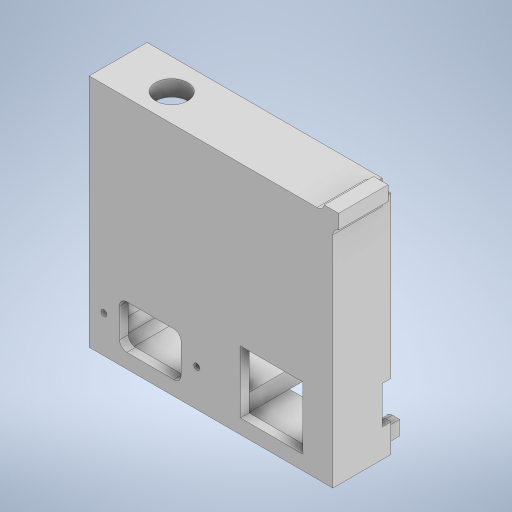
# Autodesk Inventor part: bottom
Saved by Autodesk Inventor 2023 (Build 270158000, 158)
## iProperties
Created: 2022-04-19
Part Number: bottom
Material: Generic
Document SubType Name: Modeling
Designer: cooki
Density: 1 g/cm^3
Appearance: Default
Author: cooki
## iProperties of the stored document bottom_3DPrint.ipt
Created: 2022-04-21
Part Number: bottom_3DPrint
Material: Generic
Document SubType Name: Modeling
Designer: cooki
Density: 1 g/cm^3
Appearance: Default
Author: cooki
Autodesk Inventor part; units mm, degrees
(part 1 of 2)
ref_plane "YZ Plane" through (0, 0, 0) normal (1, 0, 0) x (0, 1, 0)
ref_plane "XZ Plane" through (0, 0, 0) normal (0, 1, 0) x (-1, 0, 0)
ref_plane "XY Plane" through (0, 0, 0) normal (0, 0, 1) x (1, 0, 0)
sketch "Sketch1" plane through (0, 0, 0) normal (0, 0, 1) x (1, 0, 0)
  line L0 (53.34, -10.795) -> (50.8, -10.795) projected
  line L1 (50.8, -48.895) -> (50.8, -10.795) projected
  line L2 (-50.8, -48.895) -> (50.8, -48.895) projected
  line L3 (-50.8, 48.895) -> (-50.8, -48.895) projected
  line L4 (-49.3242, 48.895) -> (-50.8, 48.895) projected
  line L5 (-49.3242, 48.895) -> (-49.3242, 51.435) projected
  line L6 (-53.34, 51.435) -> (-49.3242, 51.435) projected
  line L7 (-53.34, -51.435) -> (-53.34, 51.435) projected
  line L8 (53.34, -51.435) -> (-53.34, -51.435) projected
  line L9 (53.34, -10.795) -> (53.34, -51.435) projected
  line L10 (-49.3242, 48.895) -> (50.8, 48.895)
  line L11 (-49.3242, 51.435) -> (53.34, 51.435)
  line L12 (50.8, -10.795) -> (50.8, 48.895)
  line L13 (53.34, -10.795) -> (53.34, 51.435)
  point P0 (0, 0)
  constraints: 8 end point, 2 horizontal, 2 vertical
extrude "Extrusion1" add sketch "Sketch1" along normal blind 19.05 contours L9 L8 L7 L6 L5 L4 L3 L2 L1 L0 | L0 L12 L10 L5 L11 L13
sketch "Sketch2" plane through (0, 0, 19.05) normal (0, 0, 1) x (1, 0, 0)
  line L0 (-53.34, 51.435) -> (-53.34, -51.435) projected
  line L1 (-53.34, -51.435) -> (53.34, -51.435) projected
  line L2 (-53.34, 51.435) -> (53.34, 51.435)
  line L3 (53.34, 51.435) -> (53.34, -51.435)
  line L4 (53.34, -51.435) -> (-53.34, -51.435)
  line L5 (-53.34, -51.435) -> (-53.34, 51.435)
  point P0 (0, 0)
  constraints: 8 end point, 2 parallel, 1 horizontal, 1 perpendicular
extrude "Extrusion2" add sketch "Sketch2" along normal blind 3.81
sketch "Sketch3" plane through (0, 0, 22.86) normal (0, 0, 1) x (1, 0, 0)
  line L0 (49.53, -22.225) -> (-49.53, -22.225) projected
  line L1 (0, -22.225) -> (0, -48.895)
  line L2 (50.8, -48.895) -> (-50.8, -48.895) projected
  line L3 (0, -35.56) -> (53.34, -35.56)
  line L4 (53.34, -51.435) -> (53.34, 51.435) projected
  line L5 (26.67, -35.56) -> (26.67, -45.085)
  line L6 (26.67, -45.085) -> (36.83, -45.085)
  line L7 (40.005, -45.085) -> (16.256, -45.085)
  line L8 (13.081, -41.91) -> (13.081, -29.083)
  line L9 (16.256, -25.908) -> (36.83, -25.908)
  line L10 (40.005, -29.083) -> (40.005, -41.91)
  arc A0 (36.83, -45.085) -> (40.005, -41.91) centre (36.83, -41.91) ccw
  arc A1 (13.081, -41.91) -> (16.256, -45.085) centre (16.256, -41.91) ccw
  arc A2 (40.005, -29.083) -> (36.83, -25.908) centre (36.83, -29.083) ccw
  arc A3 (16.256, -25.908) -> (13.081, -29.083) centre (16.256, -29.083) ccw
  line L11 (-26.67, -45.085) -> (-36.83, -45.085)
  line L12 (-40.005, -45.085) -> (-16.256, -45.085)
  line L13 (-13.081, -41.91) -> (-13.081, -29.083)
  line L14 (-16.256, -25.908) -> (-36.83, -25.908)
  line L15 (-40.005, -29.083) -> (-40.005, -41.91)
  arc A4 (-40.005, -41.91) -> (-36.83, -45.085) centre (-36.83, -41.91) ccw
  arc A5 (-16.256, -45.085) -> (-13.081, -41.91) centre (-16.256, -41.91) ccw
  arc A6 (-36.83, -25.908) -> (-40.005, -29.083) centre (-36.83, -29.083) ccw
  arc A7 (-13.081, -29.083) -> (-16.256, -25.908) centre (-16.256, -29.083) ccw
  point P0 (0, 0)
  point P1 (13.081, -25.908)
  point P2 (13.081, -45.085)
  point P3 (40.005, -25.908)
  dimension "d4" = 9.525
  dimension "d5" = 13.335
  dimension "d6" = 26.924
  dimension "d7" = 19.177
  dimension "d8" = 3.175
  constraints: 26 end point, 16 point on circle, 14 symmetric about line, 11 point on line, 8 centre point, 8 tangent, 4 midpoint, 3 equal radius, 2 horizontal, 2 parallel, 2 perpendicular, 1 vertical, 4 other
  measures "d4" distance of L5.start L5.end
  measures "d5" distance of L5.end L7.start
  measures "d6" distance of point (13.081, -25.908) point (40.005, -25.908)
  measures "d7" distance of point (13.081, -45.085) point (13.081, -25.908)
  measures "d8" radius of A0
extrude "Extrusion3" cut sketch "Sketch3" against normal blind 3.81
sketch "Sketch4" plane through (0, 0, 22.86) normal (0, 0, 1) x (1, 0, 0)
  line L0 (50.8, -48.895) -> (50.8, 48.895)
  line L1 (50.8, 48.895) -> (-50.8, 48.895)
  line L2 (-50.8, 48.895) -> (-50.8, -48.895)
  line L3 (-50.8, -48.895) -> (50.8, -48.895)
  line L4 (-16.256, -45.085) -> (-36.83, -45.085)
  arc A0 (-40.005, -41.91) -> (-36.83, -45.085) centre (-36.83, -41.91) ccw
  line L5 (-40.005, -41.91) -> (-40.005, -29.083)
  arc A1 (-36.83, -25.908) -> (-40.005, -29.083) centre (-36.83, -29.083) ccw
  line L6 (-36.83, -25.908) -> (-16.256, -25.908)
  arc A2 (-13.081, -29.083) -> (-16.256, -25.908) centre (-16.256, -29.083) ccw
  line L7 (-13.081, -29.083) -> (-13.081, -41.91)
  arc A3 (-16.256, -45.085) -> (-13.081, -41.91) centre (-16.256, -41.91) ccw
  arc A4 (13.081, -41.91) -> (16.256, -45.085) centre (16.256, -41.91) ccw
  line L8 (13.081, -41.91) -> (13.081, -29.083)
  arc A5 (16.256, -25.908) -> (13.081, -29.083) centre (16.256, -29.083) ccw
  line L9 (16.256, -25.908) -> (36.83, -25.908)
  arc A6 (40.005, -29.083) -> (36.83, -25.908) centre (36.83, -29.083) ccw
  line L10 (40.005, -29.083) -> (40.005, -41.91)
  arc A7 (36.83, -45.085) -> (40.005, -41.91) centre (36.83, -41.91) ccw
  line L11 (36.83, -45.085) -> (16.256, -45.085)
  line L12 (53.34, 51.435) -> (-53.34, 51.435)
  line L13 (-53.34, 51.435) -> (-53.34, -51.435)
  line L14 (-53.34, -51.435) -> (53.34, -51.435)
  line L15 (53.34, -51.435) -> (53.34, 51.435)
  line L16 (26.543, -35.179) -> (6.223, -35.179)
  line L17 (6.223, -35.179) -> (46.863, -35.179)
  line L18 (50.8, -48.895) -> (-50.8, -48.895)
  line L19 (0, -48.895) -> (0, -20.9574)
  circle A8 centre (6.223, -35.179) radius 1.27
  circle A9 centre (46.863, -35.179) radius 1.27
  circle A10 centre (-6.223, -35.179) radius 1.27
  circle A11 centre (-46.863, -35.179) radius 1.27
  spline S0 degree 3 poles (5.1978, -26.6049) (5.0531, -26.6049) (4.9129, -26.5796) (4.651, -26.4704) (4.5374, -26.3925) (4.3198, -26.1853) (4.2361, -26.0666) (4.1512, -25.8725) (4.1298, -25.8046) (4.101, -25.6619) (4.0942, -25.5884) (4.0942, -25.5145) knots 0 0 0 0 0.236242 0.236242 0.463278 0.463278 0.726641 0.726641 0.861093 0.861093 1 1 1 1
  spline S1 degree 3 poles (4.0942, -25.5145) (4.0942, -25.3737) (4.1187, -25.2372) (4.2245, -24.9834) (4.2996, -24.8739) (4.4749, -24.6902) (4.597, -24.585) (4.8289, -24.4831) (4.899, -24.4609) (5.046, -24.4311) (5.1217, -24.424) (5.1978, -24.424) knots 0 0 0 0 0.28445 0.28445 0.555633 0.555633 0.797647 0.797647 0.897296 0.897296 1 1 1 1
  spline S2 degree 3 poles (5.1978, -24.424) (5.3475, -24.424) (5.4929, -24.4496) (5.7606, -24.561) (5.875, -24.6392) (6.0718, -24.8281) (6.1657, -24.9455) (6.2583, -25.1585) (6.2794, -25.226) (6.3079, -25.3679) (6.3146, -25.441) (6.3146, -25.5145) knots 0 0 0 0 0.276403 0.276403 0.535347 0.535347 0.780114 0.780114 0.888262 0.888262 1 1 1 1
  spline S3 degree 3 poles (6.3146, -25.5145) (6.3146, -25.6552) (6.2901, -25.7917) (6.1843, -26.0455) (6.1092, -26.1551) (5.9462, -26.326) (5.8257, -26.4366) (5.5805, -26.5444) (5.5081, -26.567) (5.3558, -26.5978) (5.277, -26.6049) (5.1978, -26.6049) knots 0 0 0 0 0.306185 0.306185 0.598089 0.598089 0.819962 0.819962 0.908282 0.908282 1 1 1 1
  spline S4 degree 3 poles (9.8618, -39.2173) (9.7254, -39.2173) (9.5913, -39.1958) (9.33, -39.0883) (9.2363, -39.0116) (9.0945, -38.8721) (9.0324, -38.7816) (8.9368, -38.5537) (8.9159, -38.4198) (8.9159, -38.2846) knots 0 0 0 0 0.195595 0.195595 0.405153 0.405153 0.67435 0.67435 1 1 1 1
  spline S5 degree 3 poles (8.9159, -38.2846) (8.9159, -37.4855) (9.0782, -36.5199) (9.2325, -35.5792) (9.3231, -34.8494) (9.3231, -34.2512) knots 0 0 0 0 0.239723 0.239723 0.894859 0.894859 0.894859 0.894859
  line L20 (9.3231, -34.2512) -> (9.31, -33.371)
  line L21 (9.31, -33.371) -> (9.31, -32.425)
  spline S6 degree 3 poles (9.31, -32.425) (9.3214, -31.9255) (9.3575, -31.3944) (9.5041, -30.5323) (9.6012, -30.1386) (9.7567, -29.7974) knots 0 0 0 0 0.572323 0.572323 1 1 1 1
  spline S7 degree 3 poles (9.7567, -29.7974) (9.8824, -29.5153) (10.0496, -29.255) (10.4599, -28.8616) (10.6752, -28.7258) (11.2164, -28.5155) (11.5377, -28.4705) (11.8588, -28.4705) knots 0 0 0 0 0.34729 0.34729 0.638954 0.638954 1 1 1 1
  spline S8 degree 3 poles (11.8588, -28.4705) (12.2099, -28.4705) (12.5487, -28.5408) (13.2841, -28.8321) (13.657, -29.0802) (14.4056, -29.7206) (14.7781, -30.1487) (15.1038, -30.5857) knots 0 0 0 0 0.262666 0.262666 0.591662 0.591662 1 1 1 1
  line L22 (15.1038, -30.5857) -> (15.1301, -29.4821)
  spline S9 degree 3 poles (15.1301, -29.4821) (15.1473, -29.2515) (15.1886, -29.0015) (15.3312, -28.672) (15.3984, -28.5628) (15.5607, -28.4025) (15.6433, -28.3479) (15.8489, -28.2651) (15.9686, -28.2472) (16.0892, -28.2472) knots 0 0 0 0 0.399692 0.399692 0.618402 0.618402 0.792341 0.792341 1 1 1 1
  spline S10 degree 3 poles (16.0892, -28.2472) (16.221, -28.2472) (16.3498, -28.2687) (16.6015, -28.3727) (16.6969, -28.4489) (16.8417, -28.5901) (16.9052, -28.6808) (16.9741, -28.8429) (16.992, -28.9033) (17.0164, -29.0319) (17.022, -29.0993) (17.022, -29.1668) knots 0 0 0 0 0.201212 0.201212 0.415858 0.415858 0.686307 0.686307 0.838093 0.838093 1 1 1 1
  spline S11 degree 3 poles (17.022, -29.1668) (17.022, -29.4784) (16.9959, -29.9443) (16.9753, -30.3191) (16.9563, -30.7049) (16.9563, -30.9667) knots 0 0 0 0 0.326745 0.326745 1 1 1 1
  spline S12 degree 3 poles (16.9563, -30.9667) (16.9563, -31.9695) (17.0606, -33.3007) (17.1487, -34.4506) (17.219, -35.5256) (17.219, -36.3401) knots 0 0 0 0 0.30083 0.30083 0.980723 0.980723 0.980723 0.980723
  spline S13 degree 3 poles (17.219, -36.3401) (17.219, -36.6382) (17.172, -37.0783) (17.1299, -37.4813) (17.1008, -37.8136) (17.1008, -38.0481) knots 0 0 0 0 0.287253 0.287253 1 1 1 1
  spline S14 degree 3 poles (17.1008, -38.0481) (17.1008, -38.1867) (17.0799, -38.3241) (16.9761, -38.579) (16.9052, -38.6703) (16.7594, -38.8172) (16.6678, -38.8798) (16.442, -38.9735) (16.3125, -38.994) (16.1811, -38.994) knots 0 0 0 0 0.220047 0.220047 0.436643 0.436643 0.697196 0.697196 1 1 1 1
  spline S15 degree 3 poles (16.1811, -38.994) (16.0491, -38.994) (15.9191, -38.9733) (15.6914, -38.8797) (15.5984, -38.8171) (15.452, -38.6732) (15.3779, -38.5821) (15.2701, -38.3255) (15.2484, -38.1876) (15.2484, -38.0481) knots 0 0 0 0 0.307889 0.307889 0.573995 0.573995 0.786391 0.786391 1 1 1 1
  spline S16 degree 3 poles (15.2484, -38.0481) (15.2484, -37.7503) (15.2953, -37.3108) (15.3369, -36.9133) (15.3666, -36.5797) (15.3666, -36.3533) knots 0 0 0 0 0.293522 0.293522 1 1 1 1
  spline S17 degree 3 poles (15.3666, -36.3533) (15.3666, -36.2021) (15.3621, -36.0509) (15.3446, -35.7442) (15.3313, -35.5887) (15.314, -35.4336) knots 0 0 0 0 0.492094 0.492094 1 1 1 1
  spline S18 degree 3 poles (15.314, -35.4336) (15.2942, -35.267) (15.2749, -35.0948) (15.2447, -34.7923) (15.2318, -34.65) (15.2221, -34.514) knots 0 0 0 0 0.552069 0.552069 1 1 1 1
  spline S19 degree 3 poles (15.2221, -34.514) (15.0706, -33.9694) (14.8804, -33.4297) (14.4273, -32.4619) (14.1731, -32.0246) (13.8689, -31.6236) knots 0 0 0 0 0.529065 0.529065 1 1 1 1
  spline S20 degree 3 poles (13.8689, -31.6236) (13.5955, -31.2679) (13.2661, -30.9235) (12.7228, -30.5884) (12.552, -30.5079) (12.1997, -30.402) (12.0246, -30.3755) (11.8456, -30.3755) knots 0 0 0 0 0.549962 0.549962 0.781031 0.781031 1 1 1 1
  spline S21 degree 3 poles (11.8456, -30.3755) (11.7814, -30.3755) (11.7191, -30.3868) (11.6028, -30.4353) (11.5523, -30.4699) (11.4466, -30.5705) (11.3977, -30.642) (11.2805, -30.8628) (11.2298, -31.0383) (11.1205, -31.5584) (11.0968, -31.9916) (11.0968, -32.4119) knots 0 0 0 0 0.086394 0.086394 0.1694 0.1694 0.282571 0.282571 0.505651 0.505651 1 1 1 1
  spline S22 degree 3 poles (11.0968, -32.4119) (11.0968, -32.6828) (11.1229, -33.1765) (11.144, -33.5816) (11.1625, -33.9721) (11.1625, -34.1987) knots 0 0 0 0 0.31783 0.31783 1 1 1 1
  spline S23 degree 3 poles (11.1625, -34.1987) (11.1625, -34.5302) (11.1507, -34.863) (11.1069, -35.55) (11.0733, -35.9069) (11.0311, -36.2613) knots 0 0 0 0 0.481562 0.481562 1 1 1 1
  line L23 (11.0311, -36.2613) -> (10.7683, -38.3371)
  spline S24 degree 3 poles (10.7683, -38.3371) (10.7498, -38.4922) (10.7122, -38.6512) (10.5931, -38.882) (10.5316, -38.9637) (10.3807, -39.0911) (10.299, -39.1354) (10.0983, -39.2031) (9.9793, -39.2173) (9.8618, -39.2173) knots 0 0 0 0 0.331706 0.331706 0.550792 0.550792 0.750624 0.750624 1 1 1 1
  spline S25 degree 3 poles (23.2756, -38.9809) (22.808, -38.9809) (22.3454, -38.9243) (21.3996, -38.7077) (20.9233, -38.5416) (20.4641, -38.3371) knots 0 0 0 0 0.481941 0.481941 1 1 1 1
  spline S26 degree 3 poles (20.4641, -38.3371) (19.9578, -38.1116) (19.516, -37.8437) (19.0799, -37.3829) (18.9668, -37.2256) (18.8546, -36.9682) (18.8275, -36.8845) (18.7913, -36.712) (18.7825, -36.6251) (18.7825, -36.5372) knots 0 0 0 0 0.545368 0.545368 0.782666 0.782666 0.891644 0.891644 1 1 1 1
  spline S27 degree 3 poles (18.7825, -36.5372) (18.7825, -36.4354) (18.8009, -36.3371) (18.8794, -36.1493) (18.9368, -36.066) (19.0668, -35.9277) (19.1631, -35.8403) (19.3452, -35.7568) (19.3984, -35.7391) (19.5094, -35.7152) (19.5661, -35.7095) (19.6233, -35.7095) knots 0 0 0 0 0.281868 0.281868 0.563525 0.563525 0.807558 0.807558 0.903088 0.903088 1 1 1 1
  spline S28 degree 3 poles (19.6233, -35.7095) (19.6941, -35.7095) (19.7623, -35.7236) (19.9064, -35.7818) (19.9775, -35.8297) (20.1871, -36.0132) (20.285, -36.174) (20.3999, -36.3453) (20.4978, -36.4402) (20.8815, -36.7319) (21.2797, -36.8956) (21.7516, -37.0233) knots 0 0 0 0 0.043235 0.043235 0.09489 0.09489 0.213394 0.213394 0.43144 0.43144 1 1 1 1
  spline S29 degree 3 poles (21.7516, -37.0233) (22.0177, -37.0999) (22.2928, -37.1658) (22.7993, -37.2487) (23.0394, -37.2729) (23.2756, -37.2729) knots 0 0 0 0 0.539774 0.539774 1 1 1 1
  spline S30 degree 3 poles (23.2756, -37.2729) (23.8206, -37.2729) (24.3617, -37.1914) (25.1792, -36.8578) (25.4668, -36.6869) (25.9949, -36.2475) (26.2224, -35.9862) (26.4156, -35.6964) knots 0 0 0 0 0.443132 0.443132 0.717668 0.717668 1 1 1 1
  line L24 (26.4156, -35.6964) -> (22.8158, -33.9884)
  spline S31 degree 3 poles (22.8158, -33.9884) (22.4136, -33.8012) (21.9495, -33.5788) (21.2988, -33.2363) (21.0099, -33.0754) (20.8188, -32.9374) knots 0 0 0 0 0.60689 0.60689 1 1 1 1
  spline S32 degree 3 poles (20.8188, -32.9374) (20.5122, -32.7141) (20.2205, -32.4427) (19.9352, -31.9814) (19.8671, -31.8345) (19.7767, -31.5278) (19.7547, -31.3736) (19.7547, -31.2163) knots 0 0 0 0 0.542953 0.542953 0.77521 0.77521 1 1 1 1
  spline S33 degree 3 poles (19.7547, -31.2163) (19.7547, -30.9106) (19.8024, -30.6094) (20.0184, -30.0832) (20.1625, -29.8689) (20.5307, -29.4948) (20.746, -29.3433) (20.9765, -29.2194) knots 0 0 0 0 0.368171 0.368171 0.684871 0.684871 1 1 1 1
  spline S34 degree 3 poles (20.9765, -29.2194) (21.3295, -29.0311) (21.7146, -28.906) (22.5691, -28.7298) (23.053, -28.6939) (23.5252, -28.6939) knots 0 0 0 0 0.458426 0.458426 1 1 1 1
  spline S35 degree 3 poles (23.5252, -28.6939) (24.0872, -28.6939) (24.6359, -28.7863) (25.5139, -29.15) (25.8421, -29.3502) (26.4615, -29.8611) (26.7389, -30.1701) (26.9805, -30.5069) knots 0 0 0 0 0.41174 0.41174 0.696284 0.696284 1 1 1 1
  spline S36 degree 3 poles (26.9805, -30.5069) (27.3845, -31.0725) (27.6753, -31.6946) (28.0778, -33.0945) (28.1629, -33.8577) (28.1629, -34.6191) knots 0 0 0 0 0.477186 0.477186 1 1 1 1
  spline S37 degree 3 poles (28.1629, -34.6191) (28.1629, -35.2407) (28.0693, -35.8584) (27.7114, -36.7202) (27.559, -36.9889) (27.1824, -37.491) (26.9626, -37.7163) (26.7178, -37.9167) knots 0 0 0 0 0.497647 0.497647 0.746783 0.746783 1 1 1 1
  spline S38 degree 3 poles (26.7178, -37.9167) (26.2742, -38.276) (25.7739, -38.5338) (24.6006, -38.9043) (23.935, -38.9809) (23.2756, -38.9809) knots 0 0 0 0 0.463892 0.463892 1 1 1 1
  spline S39 degree 3 poles (24.55, 7.0628) (24.3391, 7.0628) (24.1103, 7.083) (23.795, 7.1882) (23.6858, 7.2429) (23.5211, 7.3827) (23.463, 7.4558) (23.3881, 7.6032) (23.3658, 7.6694) (23.3349, 7.8138) (23.3282, 7.8918) (23.3282, 7.9693) knots 0 0 0 0 0.367887 0.367887 0.577917 0.577917 0.743409 0.743409 0.865236 0.865236 1 1 1 1
  spline S40 degree 3 poles (23.3282, 7.9693) (23.3282, 8.0873) (23.3454, 8.2049) (23.4252, 8.4025) (23.4764, 8.4804) (23.6148, 8.6203) (23.7, 8.6763) (23.9128, 8.7773) (24.0467, 8.8137) (24.3423, 8.8655) (24.5152, 8.8758) (24.6814, 8.8758) knots 0 0 0 0 0.191837 0.191837 0.346324 0.346324 0.511677 0.511677 0.729348 0.729348 1 1 1 1
  spline S41 degree 3 poles (24.6814, 8.8758) (25.2902, 8.8758) (25.9168, 8.7986) (26.7317, 8.4804) (26.9656, 8.3573) (27.3917, 8.0536) (27.5785, 7.8792) (27.7425, 7.6802) knots 0 0 0 0 0.53812 0.53812 0.772375 0.772375 1 1 1 1
  spline S42 degree 3 poles (27.7425, 7.6802) (28.006, 7.3573) (28.2015, 6.9763) (28.5856, 5.9606) (28.7184, 5.2567) (28.7936, 4.5928) knots 0 0 0 0 0.383516 0.383516 1 1 1 1
  spline S43 degree 3 poles (28.7936, 4.5928) (28.8281, 4.3278) (28.8619, 4.0478) (28.909, 3.5816) (28.928, 3.3621) (28.9381, 3.1608) knots 0 0 0 0 0.571065 0.571065 1 1 1 1
  line L25 (28.9381, 3.1608) -> (29.8446, 3.1345)
  spline S44 degree 3 poles (29.8446, 3.1345) (30.2135, 3.1228) (30.5883, 3.0764) (31.0202, 2.9059) (31.1484, 2.8354) (31.3272, 2.6697) (31.3869, 2.5899) (31.4532, 2.4448) (31.4707, 2.3897) (31.4945, 2.2724) (31.5, 2.2108) (31.5, 2.1492) knots 0 0 0 0 0.470053 0.470053 0.677552 0.677552 0.825406 0.825406 0.910068 0.910068 1 1 1 1
  spline S45 degree 3 poles (31.5, 2.1492) (31.5, 2.0093) (31.4828, 1.8648) (31.3995, 1.6452) (31.3518, 1.5647) (31.2261, 1.4316) (31.1545, 1.3817) (30.9986, 1.3078) (30.9171, 1.2836) (30.7384, 1.2497) (30.6387, 1.2427) (30.5409, 1.2427) knots 0 0 0 0 0.277245 0.277245 0.464887 0.464887 0.639783 0.639783 0.80628 0.80628 1 1 1 1
  spline S46 degree 3 poles (30.5409, 1.2427) (30.4096, 1.2427) (30.1775, 1.2558) (29.718, 1.2843) (29.3538, 1.3115) (29.0563, 1.3346) knots 0 0 0 0 0.345653 0.345653 1 1 1 1
  line L26 (29.0563, 1.3346) -> (29.0563, -1.3981)
  line L27 (29.0563, -1.3981) -> (29.03, -3.96)
  spline S47 degree 3 poles (29.03, -3.96) (29.03, -4.4228) (29.0452, -4.8877) (29.1109, -5.7765) (29.1589, -6.2041) (29.2271, -6.627) knots 0 0 0 0 0.519378 0.519378 1 1 1 1
  spline S48 degree 3 poles (29.2271, -6.627) (29.2309, -6.6612) (29.2345, -6.6977) (29.2388, -6.7573) (29.2402, -6.7855) (29.2402, -6.8109) knots 0 0 0 0 0.576715 0.576715 1 1 1 1
  spline S49 degree 3 poles (29.2402, -6.8109) (29.2402, -6.928) (29.2212, -7.0425) (29.1364, -7.2475) (29.0786, -7.3327) (28.9316, -7.4837) (28.8363, -7.5568) (28.6556, -7.6369) (28.5904, -7.6572) (28.4521, -7.6848) (28.3799, -7.6911) (28.3075, -7.6911) knots 0 0 0 0 0.263935 0.263935 0.499886 0.499886 0.738828 0.738828 0.865861 0.865861 1 1 1 1
  spline S50 degree 3 poles (28.3075, -7.6911) (28.1822, -7.6911) (28.0563, -7.6736) (27.8506, -7.5915) (27.7712, -7.5405) (27.636, -7.4078) (27.5835, -7.331) (27.4948, -7.1514) (27.4624, -7.047) (27.4404, -6.9423) knots 0 0 0 0 0.297055 0.297055 0.525046 0.525046 0.746157 0.746157 1 1 1 1
  spline S51 degree 3 poles (27.4404, -6.9423) (27.3597, -6.559) (27.3119, -6.1329) (27.2435, -5.2211) (27.2301, -4.667) (27.2301, -4.1439) knots 0 0 0 0 0.427105 0.427105 1 1 1 1
  spline S52 degree 3 poles (27.2301, -4.1439) (27.2301, -3.5608) (27.2616, -2.6471) (27.2862, -1.9156) (27.309, -1.1612) (27.309, -0.6492) knots 0 0 0 0 0.174921 0.174921 0.538921 0.538921 0.538921 0.538921
  line L28 (27.309, -0.6492) -> (27.2301, 1.4923)
  spline S53 degree 3 poles (27.2301, 1.4923) (26.6512, 1.5402) (25.6364, 1.6415) (24.8138, 1.6162) (24.5529, 1.6232) (24.3135, 1.6631) knots 0 0 0 0 0.705808 0.705808 1 1 1 1
  spline S54 degree 3 poles (24.3135, 1.6631) (24.179, 1.6871) (24.0432, 1.7285) (23.8459, 1.8469) (23.7764, 1.9071) (23.6692, 2.0524) (23.6331, 2.1309) (23.587, 2.3004) (23.5778, 2.3893) (23.5778, 2.4776) knots 0 0 0 0 0.337264 0.337264 0.56702 0.56702 0.782375 0.782375 1 1 1 1
  spline S55 degree 3 poles (23.5778, 2.4776) (23.5778, 2.5965) (23.5955, 2.7145) (23.6775, 2.9161) (23.7311, 2.9967) (23.8768, 3.1432) (23.9675, 3.2025) (24.201, 3.3136) (24.3528, 3.3542) (24.688, 3.4122) (24.886, 3.4235) (25.0755, 3.4235) knots 0 0 0 0 0.178478 0.178478 0.326633 0.326633 0.488607 0.488607 0.714864 0.714864 1 1 1 1
  spline S56 degree 3 poles (25.0755, 3.4235) (25.2694, 3.4235) (25.5805, 3.4078) (26.2353, 3.3702) (26.7277, 3.3356) (27.1382, 3.3053) knots 0 0 0 0 0.367435 0.367435 1 1 1 1
  line L29 (27.1382, 3.3053) -> (27.1119, 3.8965)
  spline S57 degree 3 poles (27.1119, 3.8965) (27.0606, 4.4848) (26.9464, 5.1167) (26.5672, 5.9617) (26.3864, 6.2452) (25.9477, 6.6659) (25.721, 6.8094) (25.1733, 7.0184) (24.8624, 7.0628) (24.55, 7.0628) knots 0 0 0 0 0.391624 0.391624 0.612461 0.612461 0.793417 0.793417 1 1 1 1
  spline S58 degree 3 poles (37.504, -6.7452) (36.9873, -6.7452) (36.4832, -6.6597) (35.6732, -6.3239) (35.369, -6.1379) (34.7942, -5.6636) (34.5363, -5.3763) (34.3115, -5.0636) knots 0 0 0 0 0.40946 0.40946 0.69478 0.69478 1 1 1 1
  spline S59 degree 3 poles (34.3115, -5.0636) (33.9524, -4.567) (33.6863, -4.0237) (33.3147, -2.8107) (33.2293, -2.1588) (33.221, -1.5032) knots 0 0 0 0 0.483072 0.483072 1 1 1 1
  spline S60 degree 3 poles (33.221, -1.5032) (33.2129, -0.8912) (33.2621, -0.2746) (33.515, 0.8615) (33.7016, 1.378) (33.9699, 1.8601) knots 0 0 0 0 0.525979 0.525979 1 1 1 1
  spline S61 degree 3 poles (33.9699, 1.8601) (34.1969, 2.2675) (34.4831, 2.6384) (35.1171, 3.1473) (35.4167, 3.31) (36.093, 3.533) (36.4552, 3.5812) (36.8208, 3.5812) knots 0 0 0 0 0.39582 0.39582 0.689768 0.689768 1 1 1 1
  spline S62 degree 3 poles (36.8208, 3.5812) (37.4273, 3.5812) (38.0235, 3.4855) (38.9638, 3.0987) (39.3103, 2.8878) (39.957, 2.3465) (40.2416, 2.0203) (40.4863, 1.6631) knots 0 0 0 0 0.418318 0.418318 0.701309 0.701309 1 1 1 1
  spline S63 degree 3 poles (40.4863, 1.6631) (40.8607, 1.1277) (41.1399, 0.5468) (41.508, -0.7324) (41.5804, -1.4036) (41.5636, -2.0812) knots 0 0 0 0 0.49077 0.49077 1 1 1 1
  spline S64 degree 3 poles (41.5636, -2.0812) (41.5435, -2.7531) (41.4365, -3.4241) (41.086, -4.3381) (40.95, -4.6114) (40.6226, -5.1247) (40.4352, -5.36) (40.2236, -5.5759) knots 0 0 0 0 0.524815 0.524815 0.764006 0.764006 1 1 1 1
  spline S65 degree 3 poles (40.2236, -5.5759) (39.8618, -5.946) (39.4477, -6.2484) (38.7443, -6.5509) (38.5085, -6.6237) (38.0142, -6.7221) (37.7599, -6.7452) (37.504, -6.7452) knots 0 0 0 0 0.506666 0.506666 0.7495 0.7495 1 1 1 1
  spline S66 degree 3 poles (4.5672, 30.2201) (4.5504, 30.4221) (4.5126, 30.7046) (4.436, 31.2491) (4.3736, 31.6475) (4.3176, 31.9937) knots 0 0 0 0 0.358819 0.358819 1 1 1 1
  spline S67 degree 3 poles (4.3176, 31.9937) (4.2599, 32.3246) (4.2064, 32.6744) (4.1421, 33.2619) (4.1205, 33.5382) (4.1205, 33.7936) knots 0 0 0 0 0.568894 0.568894 1 1 1 1
  spline S68 degree 3 poles (4.1205, 33.7936) (4.1205, 33.9728) (4.141, 34.1603) (4.2425, 34.4373) (4.2989, 34.537) (4.4467, 34.6978) (4.5289, 34.7569) (4.6957, 34.8369) (4.7743, 34.8621) (4.9456, 34.8986) (5.0393, 34.9079) (5.1321, 34.9103) knots 0 0 0 0 0.313218 0.313218 0.514842 0.514842 0.694378 0.694378 0.837813 0.837813 1 1 1 1
  spline S69 degree 3 poles (5.1321, 34.9103) (5.2489, 35.0879) (5.3965, 35.2358) (5.7182, 35.4584) (5.9348, 35.576) (6.655, 35.7793) (7.0863, 35.8169) (7.497, 35.8169) knots 0 0 0 0 0.34883 0.34883 0.642178 0.642178 1 1 1 1
  spline S70 degree 3 poles (7.497, 35.8169) (8.2914, 35.8169) (9.0852, 35.7047) (10.1639, 35.2843) (10.4845, 35.1182) (11.0863, 34.7125) (11.3603, 34.478) (11.6091, 34.214) knots 0 0 0 0 0.522663 0.522663 0.76144 0.76144 1 1 1 1
  spline S71 degree 3 poles (11.6091, 34.214) (12.0744, 33.7194) (12.4245, 33.1526) (12.9547, 31.7519) (13.0675, 30.9333) (13.0675, 30.115) knots 0 0 0 0 0.453406 0.453406 1 1 1 1
  spline S72 degree 3 poles (13.0675, 30.115) (13.0675, 29.4782) (12.9739, 28.844) (12.5039, 27.6836) (12.1857, 27.2713) (11.5574, 26.6423) (11.1789, 26.3841) (10.2609, 26.0066) (9.7437, 25.924) (9.218, 25.924) knots 0 0 0 0 0.191052 0.191052 0.37544 0.37544 0.579348 0.579348 0.808983 0.808983 0.808983 0.808983
  spline S73 degree 3 poles (9.218, 25.924) (8.8759, 25.924) (8.545, 25.9847) (7.9211, 26.245) (7.6488, 26.4328) (6.9804, 27.0642) (6.6557, 27.5878) (6.4065, 28.118) knots 0 0 0 0 0.270449 0.270449 0.534405 0.534405 1 1 1 1
  spline S74 degree 3 poles (6.4065, 28.118) (6.414, 27.4031) (6.4489, 26.6312) (6.6066, 25.4165) (6.7127, 24.8517) (6.8926, 24.3737) knots 0 0 0 0 0.584935 0.584935 1 1 1 1
  spline S75 degree 3 poles (6.8926, 24.3737) (7.0374, 23.9867) (7.2366, 23.6155) (7.7219, 23.079) (7.9646, 22.8955) (8.4147, 22.6839) (8.5923, 22.6258) (8.9728, 22.5442) (9.1741, 22.5242) (9.3757, 22.5213) knots 0 0 0 0 0.371683 0.371683 0.65023 0.65023 0.818775 0.818775 1 1 1 1
  spline S76 degree 3 poles (9.3757, 22.5213) (10.3476, 22.508) (10.9453, 22.6343) (11.6154, 22.7727) (12.0198, 22.8366) (12.266, 22.8366) knots 0 0 0 0 0.291604 0.291604 1.060019 1.060019 1.060019 1.060019
  spline S77 degree 3 poles (12.266, 22.8366) (12.3929, 22.8366) (12.5244, 22.8213) (12.7229, 22.7465) (12.7952, 22.704) (12.9143, 22.5922) (12.9588, 22.5289) (13.0238, 22.3921) (13.0449, 22.3214) (13.0744, 22.1665) (13.0806, 22.0804) (13.0806, 21.9957) knots 0 0 0 0 0.283528 0.283528 0.473153 0.473153 0.648065 0.648065 0.811084 0.811084 1 1 1 1
  spline S78 degree 3 poles (13.0806, 21.9957) (13.0806, 21.8893) (13.0627, 21.7857) (12.9842, 21.5966) (12.9295, 21.5165) (12.7735, 21.3547) (12.6664, 21.2824) (12.3535, 21.121) (12.1189, 21.0545) (11.8982, 21.0104) knots 0 0 0 0 0.191146 0.191146 0.367512 0.367512 0.594676 0.594676 1 1 1 1
  spline S79 degree 3 poles (11.8982, 21.0104) (11.587, 20.9482) (11.2617, 20.908) (10.5665, 20.8515) (10.1764, 20.8396) (9.7961, 20.8396) knots 0 0 0 0 0.454615 0.454615 1 1 1 1
  spline S80 degree 3 poles (9.7961, 20.8396) (9.1683, 20.8396) (8.5145, 20.8964) (7.409, 21.1938) (6.9322, 21.4024) (6.5248, 21.7199) knots 0 0 0 0 0.549017 0.549017 1 1 1 1
  spline S81 degree 3 poles (6.5248, 21.7199) (6.2081, 21.9651) (5.9504, 22.2683) (5.4836, 23.0264) (5.3017, 23.4945) (5.1716, 23.9664) knots 0 0 0 0 0.449811 0.449811 1 1 1 1
  spline S82 degree 3 poles (5.1716, 23.9664) (5.0506, 24.4117) (4.9672, 24.8854) (4.8371, 25.9045) (4.7972, 26.4881) (4.7774, 27.0539) knots 0 0 0 0 0.448685 0.448685 1 1 1 1
  line L30 (4.7774, 27.0539) -> (4.5672, 30.2201)
  spline S83 degree 3 poles (25.3383, 38.1029) (25.1936, 38.1029) (25.0534, 38.1282) (24.7914, 38.2374) (24.6779, 38.3153) (24.4603, 38.5225) (24.3766, 38.6412) (24.2916, 38.8353) (24.2703, 38.9032) (24.2415, 39.0458) (24.2347, 39.1193) (24.2347, 39.1933) knots 0 0 0 0 0.236242 0.236242 0.463278 0.463278 0.726641 0.726641 0.861093 0.861093 1 1 1 1
  spline S84 degree 3 poles (24.2347, 39.1933) (24.2347, 39.3341) (24.2592, 39.4705) (24.3649, 39.7244) (24.44, 39.8339) (24.6153, 40.0176) (24.7375, 40.1228) (24.9694, 40.2247) (25.0395, 40.2468) (25.1865, 40.2767) (25.2621, 40.2837) (25.3383, 40.2837) knots 0 0 0 0 0.28445 0.28445 0.555633 0.555633 0.797647 0.797647 0.897296 0.897296 1 1 1 1
  spline S85 degree 3 poles (25.3383, 40.2837) (25.488, 40.2837) (25.6334, 40.2582) (25.9011, 40.1468) (26.0154, 40.0686) (26.2123, 39.8797) (26.3062, 39.7623) (26.3988, 39.5493) (26.4198, 39.4817) (26.4483, 39.3399) (26.455, 39.2668) (26.455, 39.1933) knots 0 0 0 0 0.276403 0.276403 0.535347 0.535347 0.780114 0.780114 0.888262 0.888262 1 1 1 1
  spline S86 degree 3 poles (26.455, 39.1933) (26.455, 39.0525) (26.4305, 38.9161) (26.3248, 38.6622) (26.2497, 38.5527) (26.0866, 38.3818) (25.9661, 38.2712) (25.7209, 38.1634) (25.6486, 38.1407) (25.4962, 38.11) (25.4175, 38.1029) (25.3383, 38.1029) knots 0 0 0 0 0.306185 0.306185 0.598089 0.598089 0.819962 0.819962 0.908282 0.908282 1 1 1 1
  spline S87 degree 3 poles (32.2226, 26.2262) (31.5383, 26.6961) (30.973, 27.2826) (30.2331, 28.4175) (29.9061, 29.0305) (29.4914, 30.3982) (29.3979, 31.038) (29.3979, 31.6915) knots 0 0 0 0 0.24902 0.24902 0.40645 0.40645 0.539096 0.539096 0.539096 0.539096
  spline S88 degree 3 poles (29.3979, 31.6915) (29.3979, 32.5317) (29.5615, 33.3386) (30.2862, 35.0538) (30.8981, 35.8807) (31.6182, 36.6051) knots 0 0 0 0 0.252038 0.252038 0.558585 0.558585 0.558585 0.558585
  spline S89 degree 3 poles (31.6182, 36.6051) (32.2454, 37.2367) (32.9387, 37.785) (34.4783, 38.7301) (35.309, 39.1099) (36.1771, 39.4035) knots 0 0 0 0 0.267041 0.267041 0.541966 0.541966 0.541966 0.541966
  spline S90 degree 3 poles (36.1771, 39.4035) (36.2704, 39.4364) (36.5085, 39.5459) (37.06, 39.8045) (37.5163, 40.0252) (37.8587, 40.1918) knots 0 0 0 0 0.363788 0.363788 1 1 1 1
  spline S91 degree 3 poles (37.8587, 40.1918) (38.1593, 40.3405) (38.5589, 40.5334) (39.1164, 40.7661) (39.288, 40.8224) (39.3696, 40.8224) knots 0 0 0 0 0.564502 0.564502 1 1 1 1
  spline S92 degree 3 poles (39.3696, 40.8224) (39.4673, 40.8224) (39.5619, 40.8027) (39.7721, 40.7209) (39.8814, 40.649) (40.1257, 40.4443) (40.292, 40.2609) (40.4492, 39.9954) (40.4882, 39.9125) (40.5386, 39.7484) (40.552, 39.6687) (40.552, 39.5874) knots 0 0 0 0 0.172306 0.172306 0.397602 0.397602 0.734613 0.734613 0.874501 0.874501 1 1 1 1
  spline S93 degree 3 poles (40.552, 39.5874) (40.552, 38.5115) (40.5146, 36.7023) (40.4866, 35.3736) (40.46, 33.9616) (40.46, 33.0053) knots 0 0 0 0 0.322795 0.322795 1.056604 1.056604 1.056604 1.056604
  spline S94 degree 3 poles (40.46, 33.0053) (40.46, 31.976) (40.5331, 30.4408) (40.5905, 29.2123) (40.644, 27.9363) (40.644, 27.0801) knots 0 0 0 0 0.308806 0.308806 0.937602 0.937602 0.937602 0.937602
  spline S95 degree 3 poles (40.644, 27.0801) (40.644, 26.9467) (40.6218, 26.8166) (40.524, 26.5809) (40.4564, 26.4817) (40.2785, 26.2977) (40.178, 26.2282) (40.0112, 26.1564) (39.952, 26.1383) (39.8273, 26.1136) (39.7628, 26.1079) (39.698, 26.1079) knots 0 0 0 0 0.250598 0.250598 0.47923 0.47923 0.731329 0.731329 0.862995 0.862995 1 1 1 1
  line L31 (39.698, 26.1079) -> (39.5929, 26.1079)
  spline S96 degree 3 poles (39.5929, 26.1079) (39.3919, 25.9559) (39.1558, 25.8355) (38.6257, 25.6183) (38.3024, 25.5243) (37.9901, 25.451) knots 0 0 0 0 0.439413 0.439413 1 1 1 1
  spline S97 degree 3 poles (37.9901, 25.451) (37.7176, 25.3819) (37.4376, 25.3233) (36.9178, 25.249) (36.6706, 25.2277) (36.4267, 25.2277) knots 0 0 0 0 0.535653 0.535653 1 1 1 1
  spline S98 degree 3 poles (36.4267, 25.2277) (35.6242, 25.2277) (34.7845, 25.2916) (33.3741, 25.6266) (32.7561, 25.8609) (32.2226, 26.2262) knots 0 0 0 0 0.554268 0.554268 1 1 1 1
  spline S99 degree 3 poles (24.9047, 30.4434) (24.9047, 31.3517) (24.8318, 32.3756) (24.7647, 33.3443) (24.7208, 34.1579) (24.7208, 34.8578) knots 0 0 0 0 0.272485 0.272485 0.959703 0.959703 0.959703 0.959703
  spline S100 degree 3 poles (24.7208, 34.8578) (24.7208, 34.9985) (24.7416, 35.1385) (24.838, 35.3763) (24.9007, 35.471) (25.0435, 35.6142) (25.134, 35.6891) (25.3178, 35.768) (25.3783, 35.7863) (25.5065, 35.8111) (25.5734, 35.8169) (25.6405, 35.8169) knots 0 0 0 0 0.330742 0.330742 0.602976 0.602976 0.805847 0.805847 0.900295 0.900295 1 1 1 1
  spline S101 degree 3 poles (25.6405, 35.8169) (25.7725, 35.8169) (25.9025, 35.7961) (26.1302, 35.7025) (26.2232, 35.6399) (26.3632, 35.5023) (26.4394, 35.4125) (26.5514, 35.1458) (26.5732, 35.0022) (26.5732, 34.8578) knots 0 0 0 0 0.321921 0.321921 0.600153 0.600153 0.800262 0.800262 1 1 1 1
  spline S102 degree 3 poles (26.5732, 34.8578) (26.5732, 33.9495) (26.6462, 32.9256) (26.7133, 31.957) (26.7572, 31.1433) (26.7572, 30.4434) knots 0 0 0 0 0.272485 0.272485 0.959703 0.959703 0.959703 0.959703
  spline S103 degree 3 poles (26.7572, 30.4434) (26.7572, 29.8609) (26.7311, 28.98) (26.7106, 28.276) (26.6915, 27.5446) (26.6915, 27.0539) knots 0 0 0 0 0.174763 0.174763 0.53175 0.53175 0.53175 0.53175
  spline S104 degree 3 poles (26.6915, 27.0539) (26.6915, 26.9174) (26.6707, 26.7824) (26.5756, 26.5495) (26.5129, 26.4557) (26.3606, 26.3018) (26.2663, 26.2297) (26.0212, 26.1287) (25.891, 26.1079) (25.7587, 26.1079) knots 0 0 0 0 0.300477 0.300477 0.553693 0.553693 0.777141 0.777141 1 1 1 1
  spline S105 degree 3 poles (25.7587, 26.1079) (25.6286, 26.1079) (25.5003, 26.128) (25.2773, 26.2194) (25.1868, 26.2801) (25.0226, 26.4421) (24.9596, 26.5362) (24.8608, 26.7724) (24.839, 26.9124) (24.839, 27.0539) knots 0 0 0 0 0.255734 0.255734 0.473941 0.473941 0.709302 0.709302 1 1 1 1
  spline S106 degree 3 poles (24.839, 27.0539) (24.839, 27.6364) (24.8652, 28.5173) (24.8856, 29.2213) (24.9047, 29.9527) (24.9047, 30.4434) knots 0 0 0 0 0.174763 0.174763 0.53175 0.53175 0.53175 0.53175
  spline S107 degree 3 poles (15.3535, 33.4126) (15.2214, 33.4126) (15.0914, 33.4333) (14.8637, 33.5269) (14.7707, 33.5895) (14.6243, 33.7334) (14.5502, 33.8245) (14.4424, 34.0811) (14.4207, 34.219) (14.4207, 34.3585) knots 0 0 0 0 0.307889 0.307889 0.573995 0.573995 0.786391 0.786391 1 1 1 1
  spline S108 degree 3 poles (14.4207, 34.3585) (14.4207, 34.5598) (14.4676, 34.8317) (14.5628, 35.282) (14.6571, 35.6899) (14.6571, 35.9745) knots 0 0 0 0 0.532399 0.532399 1 1 1 1
  spline S109 degree 3 poles (14.6571, 35.9745) (14.6571, 36.111) (14.6779, 36.246) (14.773, 36.4789) (14.8357, 36.5727) (14.9881, 36.7265) (15.0823, 36.7987) (15.3274, 36.8996) (15.4576, 36.9204) (15.5899, 36.9204) knots 0 0 0 0 0.300477 0.300477 0.553693 0.553693 0.777141 0.777141 1 1 1 1
  spline S110 degree 3 poles (15.5899, 36.9204) (15.7358, 36.9204) (15.8805, 36.9068) (16.1637, 36.8493) (16.2995, 36.8065) (16.4308, 36.7496) knots 0 0 0 0 0.504814 0.504814 1 1 1 1
  spline S111 degree 3 poles (16.4308, 36.7496) (16.9868, 36.492) (17.9543, 36.2224) (18.8181, 35.9789) (19.5406, 35.7566) (20.0043, 35.541) knots 0 0 0 0 0.183857 0.183857 0.634982 0.634982 0.634982 0.634982
  spline S112 degree 3 poles (20.0043, 35.541) (20.4132, 35.3566) (20.796, 35.1136) (21.3522, 34.534) (21.5398, 34.2414) (21.8116, 33.538) (21.8699, 33.142) (21.8699, 32.7426) knots 0 0 0 0 0.373073 0.373073 0.667821 0.667821 1 1 1 1
  spline S113 degree 3 poles (21.8699, 32.7426) (21.8699, 32.4537) (21.8278, 32.165) (21.6561, 31.746) (21.5742, 31.606) (21.3667, 31.3483) (21.2443, 31.2362) (21.1079, 31.1397) knots 0 0 0 0 0.466226 0.466226 0.73053 0.73053 1 1 1 1
  spline S114 degree 3 poles (21.1079, 31.1397) (20.9111, 31.002) (20.6592, 30.8898) (20.0644, 30.6781) (19.6853, 30.583) (19.3342, 30.5091) knots 0 0 0 0 0.430338 0.430338 1 1 1 1
  line L32 (19.3342, 30.5091) -> (18.3489, 30.2858)
  spline S115 degree 3 poles (18.3489, 30.2858) (17.9722, 30.1916) (17.5772, 30.0499) (17.0755, 29.706) (16.9162, 29.556) (16.7179, 29.2542) (16.6595, 29.1264) (16.58, 28.847) (16.5621, 28.7) (16.5621, 28.5516) knots 0 0 0 0 0.433168 0.433168 0.676792 0.676792 0.834874 0.834874 1 1 1 1
  spline S116 degree 3 poles (16.5621, 28.5516) (16.5621, 28.4584) (16.5786, 28.3681) (16.6491, 28.199) (16.6996, 28.1254) (16.8419, 27.9756) (16.9397, 27.9069) (17.1671, 27.7814) (17.3058, 27.7273) (17.4424, 27.6845) knots 0 0 0 0 0.210328 0.210328 0.413643 0.413643 0.676539 0.676539 1 1 1 1
  spline S117 degree 3 poles (17.4424, 27.6845) (17.6517, 27.6194) (17.8689, 27.5752) (18.3333, 27.5139) (18.5858, 27.5005) (18.835, 27.5005) knots 0 0 0 0 0.467817 0.467817 1 1 1 1
  spline S118 degree 3 poles (18.835, 27.5005) (18.9943, 27.5005) (19.1596, 27.5125) (19.5108, 27.5515) (19.7084, 27.583) (19.8992, 27.6188) knots 0 0 0 0 0.450432 0.450432 1 1 1 1
  spline S119 degree 3 poles (19.8992, 27.6188) (20.1071, 27.6534) (20.3461, 27.703) (20.6195, 27.7989) (20.6956, 27.8301) (20.8159, 27.8962) (20.8687, 27.9314) (20.9108, 27.9735) knots 0 0 0 0 0.607378 0.607378 0.829871 0.829871 1 1 1 1
  spline S120 degree 3 poles (20.9108, 27.9735) (21.0333, 28.0925) (21.1805, 28.2206) (21.3833, 28.3416) (21.4433, 28.3717) (21.5543, 28.4091) (21.607, 28.4202) (21.6597, 28.4202) knots 0 0 0 0 0.5945 0.5945 0.817866 0.817866 1 1 1 1
  spline S121 degree 3 poles (21.6597, 28.4202) (21.7843, 28.4202) (21.9046, 28.3975) (22.1349, 28.3013) (22.2373, 28.2307) (22.4075, 28.0709) (22.4954, 27.9691) (22.5813, 27.7791) (22.6003, 27.7211) (22.6258, 27.5995) (22.6319, 27.5371) (22.6319, 27.4743) knots 0 0 0 0 0.277057 0.277057 0.554907 0.554907 0.796191 0.796191 0.896909 0.896909 1 1 1 1
  spline S122 degree 3 poles (22.6319, 27.4743) (22.6319, 27.3265) (22.6047, 27.184) (22.4897, 26.909) (22.4047, 26.7858) (22.1699, 26.5347) (22.0093, 26.4167) (21.6377, 26.1968) (21.4106, 26.0974) (21.1867, 26.016) knots 0 0 0 0 0.202377 0.202377 0.40818 0.40818 0.673155 0.673155 1 1 1 1
  spline S123 degree 3 poles (21.1867, 26.016) (20.8108, 25.8761) (20.4254, 25.7708) (19.6309, 25.6296) (19.2278, 25.5955) (18.8219, 25.5955) knots 0 0 0 0 0.497022 0.497022 1 1 1 1
  spline S124 degree 3 poles (18.8219, 25.5955) (18.3078, 25.5955) (17.7858, 25.6407) (16.8469, 25.8577) (16.4248, 26.0129) (16.0366, 26.2393) knots 0 0 0 0 0.533697 0.533697 1 1 1 1
  spline S125 degree 3 poles (16.0366, 26.2393) (15.7199, 26.4243) (15.436, 26.6559) (15.044, 27.1681) (14.9188, 27.4118) (14.7467, 27.9602) (14.7097, 28.255) (14.7097, 28.5516) knots 0 0 0 0 0.389669 0.389669 0.685022 0.685022 1 1 1 1
  spline S126 degree 3 poles (14.7097, 28.5516) (14.7097, 29.0228) (14.7822, 29.4881) (15.0847, 30.2269) (15.2539, 30.5017) (15.6923, 31.0101) (15.957, 31.2298) (16.2468, 31.4156) knots 0 0 0 0 0.412515 0.412515 0.698639 0.698639 1 1 1 1
  spline S127 degree 3 poles (16.2468, 31.4156) (16.6476, 31.6761) (17.1243, 31.8736) (18.1808, 32.2229) (18.8403, 32.3699) (19.4656, 32.4798) knots 0 0 0 0 0.428503 0.428503 1 1 1 1
  spline S128 degree 3 poles (19.4656, 32.4798) (19.5586, 32.4975) (19.6505, 32.5195) (19.8348, 32.5722) (19.9268, 32.6029) (20.0174, 32.6375) knots 0 0 0 0 0.493774 0.493774 1 1 1 1
  spline S129 degree 3 poles (20.0174, 32.6375) (20.0154, 32.7723) (19.9871, 32.9014) (19.874, 33.1616) (19.7871, 33.2836) (19.5448, 33.5422) (19.3728, 33.6698) (18.9774, 33.912) (18.733, 34.0262) (18.4934, 34.1221) knots 0 0 0 0 0.180216 0.180216 0.379293 0.379293 0.654194 0.654194 1 1 1 1
  spline S130 degree 3 poles (18.4934, 34.1221) (18.0835, 34.255) (17.6358, 34.3975) (16.9434, 34.6073) (16.6099, 34.7053) (16.3257, 34.779) knots 0 0 0 0 0.597182 0.597182 1 1 1 1
  spline S131 degree 3 poles (16.3257, 34.779) (16.2981, 34.5755) (16.2602, 34.3391) (16.1727, 33.9845) (16.1283, 33.8528) (16.076, 33.7673) knots 0 0 0 0 0.565724 0.565724 1 1 1 1
  spline S132 degree 3 poles (16.076, 33.7673) (16.0295, 33.6887) (15.9705, 33.621) (15.8257, 33.5131) (15.7454, 33.4759) (15.5607, 33.4233) (15.4563, 33.4126) (15.3535, 33.4126) knots 0 0 0 0 0.322337 0.322337 0.637039 0.637039 1 1 1 1
  spline S133 degree 3 poles (41.0907, -36.2088) (41.0856, -36.4806) (41.0317, -36.7423) (40.8138, -37.2379) (40.6579, -37.4555) (40.1442, -37.9804) (39.7252, -38.2341) (39.3039, -38.4291) knots 0 0 0 0 0.270178 0.270178 0.537914 0.537914 1 1 1 1
  spline S134 degree 3 poles (39.3039, -38.4291) (38.824, -38.6513) (38.3239, -38.8139) (37.2614, -39.0352) (36.7073, -39.086) (36.1508, -39.086) knots 0 0 0 0 0.487269 0.487269 1 1 1 1
  spline S135 degree 3 poles (36.1508, -39.086) (35.3984, -39.086) (34.6522, -38.9982) (33.2366, -38.6052) (32.5891, -38.3172) (31.9861, -37.9298) knots 0 0 0 0 0.51216 0.51216 1 1 1 1
  spline S136 degree 3 poles (31.9861, -37.9298) (31.4546, -37.5867) (30.9752, -37.1668) (30.3795, -36.3178) (30.2033, -35.9594) (29.9641, -35.173) (29.9103, -34.7608) (29.9103, -34.3432) knots 0 0 0 0 0.435014 0.435014 0.712932 0.712932 1 1 1 1
  spline S137 degree 3 poles (29.9103, -34.3432) (29.9103, -33.8407) (29.9954, -33.3517) (30.2834, -32.6638) (30.4002, -32.4519) (30.682, -32.044) (30.8463, -31.8526) (31.027, -31.6762) knots 0 0 0 0 0.503378 0.503378 0.747001 0.747001 1 1 1 1
  spline S138 degree 3 poles (31.027, -31.6762) (31.4179, -31.2895) (31.8725, -30.9947) (33.0129, -30.5084) (33.7026, -30.3733) (34.3903, -30.323) knots 0 0 0 0 0.443476 0.443476 1 1 1 1
  spline S139 degree 3 poles (34.3903, -30.323) (34.7854, -30.295) (35.2394, -30.2586) (35.8963, -30.1856) (36.1897, -30.147) (36.4004, -30.0996) knots 0 0 0 0 0.60247 0.60247 1 1 1 1
  spline S140 degree 3 poles (36.4004, -30.0996) (36.7801, -30.0101) (37.1232, -29.8861) (37.4886, -29.6325) (37.593, -29.5362) (37.7095, -29.3564) (37.7409, -29.2893) (37.7832, -29.1453) (37.793, -29.0713) (37.793, -28.996) knots 0 0 0 0 0.513531 0.513531 0.747902 0.747902 0.873537 0.873537 1 1 1 1
  spline S141 degree 3 poles (37.793, -28.996) (37.793, -28.7471) (37.7477, -28.5069) (37.5668, -28.0741) (37.4471, -27.8907) (37.1391, -27.538) (36.9463, -27.376) (36.742, -27.2356) knots 0 0 0 0 0.34709 0.34709 0.654152 0.654152 1 1 1 1
  spline S142 degree 3 poles (36.742, -27.2356) (36.3934, -26.9942) (36.0129, -26.8181) (35.1641, -26.5724) (34.7053, -26.5171) (34.2458, -26.513) knots 0 0 0 0 0.479885 0.479885 1 1 1 1
  spline S143 degree 3 poles (34.2458, -26.513) (33.873, -26.5036) (33.3972, -26.5772) (32.5854, -26.7418) (31.8569, -26.9071) (31.4606, -26.9071) knots 0 0 0 0 0.536395 0.536395 1 1 1 1
  spline S144 degree 3 poles (31.4606, -26.9071) (31.3273, -26.9071) (31.1884, -26.8915) (30.9814, -26.8147) (30.9066, -26.7716) (30.7847, -26.6586) (30.7397, -26.5953) (30.6752, -26.4603) (30.6546, -26.3922) (30.6258, -26.2431) (30.6197, -26.1606) (30.6197, -26.0794) knots 0 0 0 0 0.295577 0.295577 0.488885 0.488885 0.663616 0.663616 0.820056 0.820056 1 1 1 1
  spline S145 degree 3 poles (30.6197, -26.0794) (30.6197, -26.011) (30.6332, -25.9452) (30.6888, -25.8105) (30.7329, -25.7463) (30.8706, -25.5931) (30.9812, -25.5127) (31.3806, -25.2742) (31.7662, -25.1424) (32.1437, -25.0415) knots 0 0 0 0 0.11182 0.11182 0.238155 0.238155 0.448607 0.448607 1 1 1 1
  spline S146 degree 3 poles (32.1437, -25.0415) (32.502, -24.9438) (32.8703, -24.8612) (33.5567, -24.7562) (33.8834, -24.7262) (34.2064, -24.7262) knots 0 0 0 0 0.534918 0.534918 1 1 1 1
  spline S147 degree 3 poles (34.2064, -24.7262) (34.8621, -24.7262) (35.499, -24.8382) (36.7805, -25.2863) (37.3956, -25.6282) (37.9638, -26.04) knots 0 0 0 0 0.482986 0.482986 1 1 1 1
  spline S148 degree 3 poles (37.9638, -26.04) (38.5118, -26.4368) (39.0345, -26.9197) (39.5455, -27.7407) (39.6675, -28.0018) (39.8293, -28.5474) (39.8688, -28.8214) (39.8688, -29.1011) knots 0 0 0 0 0.543548 0.543548 0.775627 0.775627 1 1 1 1
  spline S149 degree 3 poles (39.8688, -29.1011) (39.8688, -29.427) (39.8158, -29.7459) (39.5801, -30.316) (39.4193, -30.553) (39.015, -30.9683) (38.7796, -31.1394) (38.5288, -31.282) knots 0 0 0 0 0.359949 0.359949 0.681301 0.681301 1 1 1 1
  spline S150 degree 3 poles (38.5288, -31.282) (38.165, -31.4912) (37.7755, -31.6432) (36.9206, -31.8647) (36.4564, -31.9225) (35.9931, -31.9389) knots 0 0 0 0 0.47507 0.47507 1 1 1 1
  spline S151 degree 3 poles (35.9931, -31.9389) (35.4766, -31.9551) (34.9534, -32.0108) (34.0101, -32.2267) (33.581, -32.3737) (33.1816, -32.5827) knots 0 0 0 0 0.534241 0.534241 1 1 1 1
  spline S152 degree 3 poles (33.1816, -32.5827) (32.8541, -32.748) (32.538, -32.9602) (32.1442, -33.404) (32.0251, -33.5928) (31.8647, -34.0153) (31.8284, -34.2355) (31.8284, -34.4614) knots 0 0 0 0 0.448365 0.448365 0.724226 0.724226 1 1 1 1
  spline S153 degree 3 poles (31.8284, -34.4614) (31.8284, -34.757) (31.8796, -35.0436) (32.1013, -35.5757) (32.2583, -35.8048) (32.7293, -36.2979) (33.074, -36.5265) (33.4312, -36.708) knots 0 0 0 0 0.302356 0.302356 0.589662 0.589662 1 1 1 1
  spline S154 degree 3 poles (33.4312, -36.708) (33.8469, -36.918) (34.2815, -37.0758) (35.2003, -37.2888) (35.6733, -37.3386) (36.1508, -37.3386) knots 0 0 0 0 0.493762 0.493762 1 1 1 1
  spline S155 degree 3 poles (36.1508, -37.3386) (36.5946, -37.3386) (37.0607, -37.3052) (37.8384, -37.1295) (38.1809, -37.0068) (38.4762, -36.8131) knots 0 0 0 0 0.557389 0.557389 1 1 1 1
  spline S156 degree 3 poles (38.4762, -36.8131) (38.6205, -36.7152) (38.7591, -36.5756) (39.0362, -36.2602) (39.193, -36.0447) (39.3302, -35.8409) knots 0 0 0 0 0.413325 0.413325 1 1 1 1
  spline S157 degree 3 poles (39.3302, -35.8409) (39.4303, -35.6926) (39.5535, -35.5507) (39.7696, -35.4081) (39.8408, -35.3731) (39.9912, -35.3266) (40.0671, -35.3154) (40.1447, -35.3154) knots 0 0 0 0 0.532387 0.532387 0.769405 0.769405 1 1 1 1
  spline S158 degree 3 poles (40.1447, -35.3154) (40.2833, -35.3154) (40.4183, -35.3385) (40.6978, -35.4545) (40.8005, -35.5426) (40.9307, -35.6708) (40.9893, -35.7541) (41.0525, -35.9044) (41.0686, -35.9614) (41.0893, -36.0824) (41.0928, -36.1456) (41.0907, -36.2088) knots 0 0 0 0 0.179682 0.179682 0.392479 0.392479 0.670408 0.670408 0.830237 0.830237 1 1 1 1
  spline S159 degree 3 poles (4.7643, -34.2643) (4.7643, -33.3561) (4.6914, -32.3322) (4.6242, -31.3635) (4.5804, -30.5498) (4.5804, -29.85) knots 0 0 0 0 0.272485 0.272485 0.959703 0.959703 0.959703 0.959703
  spline S160 degree 3 poles (4.5804, -29.85) (4.5804, -29.7093) (4.6011, -29.5693) (4.6975, -29.3314) (4.7603, -29.2368) (4.903, -29.0936) (4.9936, -29.0187) (5.1773, -28.9397) (5.2379, -28.9215) (5.3661, -28.8966) (5.4329, -28.8909) (5.5, -28.8909) knots 0 0 0 0 0.330742 0.330742 0.602976 0.602976 0.805847 0.805847 0.900295 0.900295 1 1 1 1
  spline S161 degree 3 poles (5.5, -28.8909) (5.6321, -28.8909) (5.762, -28.9116) (5.9898, -29.0052) (6.0828, -29.0679) (6.2227, -29.2054) (6.299, -29.2952) (6.4109, -29.562) (6.4328, -29.7056) (6.4328, -29.85) knots 0 0 0 0 0.321921 0.321921 0.600153 0.600153 0.800262 0.800262 1 1 1 1
  spline S162 degree 3 poles (6.4328, -29.85) (6.4328, -30.7583) (6.5057, -31.7821) (6.5728, -32.7508) (6.6167, -33.5645) (6.6167, -34.2643) knots 0 0 0 0 0.272485 0.272485 0.959703 0.959703 0.959703 0.959703
  spline S163 degree 3 poles (6.6167, -34.2643) (6.6167, -34.8469) (6.5906, -35.7277) (6.5701, -36.4318) (6.551, -37.1632) (6.551, -37.6539) knots 0 0 0 0 0.174763 0.174763 0.53175 0.53175 0.53175 0.53175
  spline S164 degree 3 poles (6.551, -37.6539) (6.551, -37.7904) (6.5303, -37.9254) (6.4352, -38.1583) (6.3725, -38.2521) (6.2201, -38.406) (6.1258, -38.4781) (5.8808, -38.5791) (5.7506, -38.5999) (5.6182, -38.5999) knots 0 0 0 0 0.300477 0.300477 0.553693 0.553693 0.777141 0.777141 1 1 1 1
  spline S165 degree 3 poles (5.6182, -38.5999) (5.4882, -38.5999) (5.3599, -38.5798) (5.1368, -38.4884) (5.0463, -38.4277) (4.8821, -38.2656) (4.8191, -38.1716) (4.7203, -37.9354) (4.6986, -37.7954) (4.6986, -37.6539) knots 0 0 0 0 0.255734 0.255734 0.473941 0.473941 0.709302 0.709302 1 1 1 1
  spline S166 degree 3 poles (4.6986, -37.6539) (4.6986, -37.0714) (4.7247, -36.1905) (4.7452, -35.4865) (4.7643, -34.7551) (4.7643, -34.2643) knots 0 0 0 0 0.174763 0.174763 0.53175 0.53175 0.53175 0.53175
  spline S167 degree 3 poles (-1.9755, -39.0991) (-2.4922, -39.0991) (-2.9963, -39.0135) (-3.8063, -38.6778) (-4.1105, -38.4918) (-4.6853, -38.0175) (-4.9432, -37.7302) (-5.168, -37.4174) knots 0 0 0 0 0.40946 0.40946 0.69478 0.69478 1 1 1 1
  spline S168 degree 3 poles (-5.168, -37.4174) (-5.5271, -36.9209) (-5.7932, -36.3776) (-6.1647, -35.1646) (-6.2502, -34.5127) (-6.2584, -33.8571) knots 0 0 0 0 0.483072 0.483072 1 1 1 1
  spline S169 degree 3 poles (-6.2584, -33.8571) (-6.2666, -33.2451) (-6.2174, -32.6285) (-5.9645, -31.4924) (-5.7779, -30.9758) (-5.5096, -30.4938) knots 0 0 0 0 0.525979 0.525979 1 1 1 1
  spline S170 degree 3 poles (-5.5096, -30.4938) (-5.2826, -30.0864) (-4.9964, -29.7155) (-4.3624, -29.2066) (-4.0628, -29.0439) (-3.3865, -28.8209) (-3.0243, -28.7727) (-2.6586, -28.7727) knots 0 0 0 0 0.39582 0.39582 0.689768 0.689768 1 1 1 1
  spline S171 degree 3 poles (-2.6586, -28.7727) (-2.0522, -28.7727) (-1.456, -28.8683) (-0.5156, -29.2552) (-0.1692, -29.4661) (0.4775, -30.0074) (0.7621, -30.3336) (1.0068, -30.6908) knots 0 0 0 0 0.418318 0.418318 0.701309 0.701309 1 1 1 1
  spline S172 degree 3 poles (1.0068, -30.6908) (1.3812, -31.2262) (1.6605, -31.8071) (2.0285, -33.0863) (2.1009, -33.7575) (2.0841, -34.4351) knots 0 0 0 0 0.49077 0.49077 1 1 1 1
  spline S173 degree 3 poles (2.0841, -34.4351) (2.064, -35.107) (1.957, -35.778) (1.6066, -36.692) (1.4706, -36.9653) (1.1431, -37.4786) (0.9557, -37.7138) (0.7441, -37.9298) knots 0 0 0 0 0.524815 0.524815 0.764006 0.764006 1 1 1 1
  spline S174 degree 3 poles (0.7441, -37.9298) (0.3823, -38.2999) (-0.0318, -38.6023) (-0.7352, -38.9048) (-0.971, -38.9776) (-1.4653, -39.076) (-1.7196, -39.0991) (-1.9755, -39.0991) knots 0 0 0 0 0.506666 0.506666 0.7495 0.7495 1 1 1 1
  point P0 (0, 0)
  dimension "d11" = 20.32
  dimension "d12" = 40.64
  dimension "d13" = 2.54
  dimension "d14" = 2.54
  constraints: 6 end point, 4 centre point, 2 coincident, 2 horizontal, 2 symmetric about line, 1 midpoint, 1 vertical, 2 other
  measures "d11" distance of L16.start L16.end
  measures "d12" distance of L16.end L17.end
  measures "d13" diameter of A8
  measures "d14" diameter of A9
extrude "Extrusion4" cut sketch "Sketch4" against normal blind 3.81 contours A8 S163 L16 | L16 S163 S162 A8 | S163 A8 S162 | S168 A10 | A10 S168 | A9 | A11